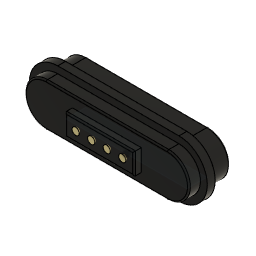
4pin_magnetic_connector_male v5 (Autodesk Fusion 360 design; units mm, degrees)
Autodesk Fusion 360 part; units mm, degrees
note: some values were not read from the file. Chosen so that the rebuilt part matches the saved one: which bodies a step acts on.
sketch "Skizze1" plane through (0, 0, 0) normal (0, 1, 0) x (1, 0, 0)
  line L0 (8.45, 3.95) -> (-8.45, 3.95)
  line L1 (-8.45, 3.95) -> (-8.45, -3.95)
  line L2 (-8.45, -3.95) -> (8.45, -3.95)
  line L3 (8.45, -3.95) -> (8.45, 3.95)
  line L4 (8.45, 3.95) -> (-8.45, -3.95) construction
  line L5 (-8.45, 3.95) -> (8.45, -3.95) construction
  arc A0 (8.45, -3.95) -> (8.45, 3.95) centre (8.45, 0) ccw
  arc A1 (-8.45, 3.95) -> (-8.45, -3.95) centre (-8.45, 0) ccw
  dimension "d1" = 16.9
  dimension "d2" = 7.9
  constraint horizontal L0
  constraint perpendicular L0 L1
  constraint parallel L0 L2
  constraint parallel L1 L3
  constraint coincident L4 origin
  constraint coincident L5 origin
  constraint midpoint L3 A0.centre
  constraint midpoint L1 A1.centre
  measures "d1" distance of L1.end L2.end
  measures "d2" distance of L0.end L1.end
extrude "Extrusion1" add sketch "Skizze1" along normal blind 1.1 makes body 1
sketch "Skizze2" plane through (0, 0, 0) normal (0, -1, 0) x (1, 0, 0)
  arc A0 (-8.45, 3.95) -> (-8.45, -3.95) centre (-8.45, 0) ccw
  line L0 (-8.45, -3.95) -> (8.45, -3.95)
  arc A1 (8.45, -3.95) -> (8.45, 3.95) centre (8.45, 0) ccw
  line L1 (8.45, 3.95) -> (-8.45, 3.95)
  arc A2 (-8.45, 3) -> (-8.45, -3) centre (-8.45, 0) ccw
  line L2 (-8.45, -3) -> (8.45, -3)
  arc A3 (8.45, -3) -> (8.45, 3) centre (8.45, 0) ccw
  line L3 (8.45, 3) -> (-8.45, 3)
  dimension "d5" = -0.95
extrude "Extrusion2" add sketch "Skizze2" along normal blind 1.6 contours A2 L2 A3 L3 bodies 1
sketch "Skizze3" plane through (0, 1.1, 0) normal (0, 1, 0) x (-1, 0, 0)
  arc A0 (8.45, -3.95) -> (8.45, 3.95) centre (8.45, 0) ccw
  line L0 (8.45, 3.95) -> (-8.45, 3.95)
  arc A1 (-8.45, 3.95) -> (-8.45, -3.95) centre (-8.45, 0) ccw
  line L1 (-8.45, -3.95) -> (8.45, -3.95)
  line L2 (-8.45, 3) -> (8.45, 3)
  arc A2 (8.45, -3) -> (8.45, 3) centre (8.45, 0) ccw
  line L3 (8.45, -3) -> (-8.45, -3)
  arc A3 (-8.45, 3) -> (-8.45, -3) centre (-8.45, 0) ccw
extrude "Extrusion3" add sketch "Skizze3" along normal blind 3 contours L2 A2 L3 A3 bodies 1
sketch "Skizze4" plane through (0, -1.6, 0) normal (0, -1, 0) x (1, 0, 0)
  line L0 (8.45, 3) -> (-8.45, 3)
  arc A0 (-8.45, 3) -> (-8.45, -3) centre (-8.45, 0) ccw
  line L1 (-8.45, -3) -> (8.45, -3)
  arc A1 (8.45, -3) -> (8.45, 3) centre (8.45, 0) ccw
  line L2 (4.8, -1.5) -> (-4.8, -1.5)
  line L3 (-4.8, -1.5) -> (-4.8, 1.5)
  line L4 (-4.8, 1.5) -> (4.8, 1.5)
  line L5 (4.8, 1.5) -> (4.8, -1.5)
  line L6 (4.8, -1.5) -> (-4.8, 1.5) construction
  line L7 (-4.8, -1.5) -> (4.8, 1.5) construction
  dimension "d10" = 9.6
  dimension "d11" = 3
  constraint horizontal L2
  constraint perpendicular L2 L3
  constraint parallel L2 L4
  constraint parallel L3 L5
  constraint coincident L6 origin
  constraint coincident L7 origin
  measures "d10" distance of L3.end L4.end
  measures "d11" distance of L2.end L3.end
extrude "Extrusion4" add sketch "Skizze4" along normal blind 1 contours L2 L3 L4 L5 bodies 1
sketch "Skizze5" plane through (0, -2.6, 0) normal (0, -1, 0) x (1, 0, 0)
  line L0 (4.8, 1.5) -> (-4.8, 1.5)
  line L1 (-4.8, 1.5) -> (-4.8, -1.5)
  line L2 (-4.8, -1.5) -> (4.8, -1.5)
  line L3 (4.8, -1.5) -> (4.8, 1.5)
  line L4 (-4.8, 0) -> (4.8, 0) construction
  circle A0 centre (-3.25, 0) radius 0.5
  circle A1 centre (-1.0833, 0) radius 0.5
  circle A2 centre (1.0833, 0) radius 0.5
  circle A3 centre (3.25, 0) radius 0.5
  line L5 (-3.25, 0) -> (-4.8, 0)
  line L6 (3.25, 0) -> (4.8, 0)
  dimension "d14" = 1
  dimension "d17" = 6.5
  dimension "d18" = 0
  constraint midpoint L1 L4.start
  constraint midpoint L3 L4.end
  constraint coincident L4 A0.centre
  constraint coincident A0.centre L5.start
  constraint perpendicular L1 L5
  constraint coincident A3.centre L6.start
  constraint perpendicular L3 L6
  constraint equal L5 L6
  measures "d14" diameter of A0
extrude "Extrusion5" add sketch "Skizze5" along normal blind 0.5 and the other way blind 8 separate body contours A0 | A1 | A2 | A3 makes body 2 at (-0.584, 2.7333, -0.0249) makes body 3 at (1.5827, 2.7333, -0.0249) makes body 4 at (-3.7494, 0.0667, -0.0249) makes body 5 at (3.7494, 2.7333, -0.0249)
fillet "Abrundung1" radius 0.2 12 edges at (0, -2.6, 1.5) (4.8, -2.6, 0) (0, -2.6, -1.5) (-4.8, -2.6, 0) (0, -1.6, -3) (11.45, -1.6, 0) (0, -1.6, 3) (-11.45, -1.6, 0) (0, 4.1, -3) (-11.45, 4.1, 0) (0, 4.1, 3) (11.45, 4.1, 0) on bodies 1
extrude "Extrusion6" cut 4 faces at (-3.1123, -3.1, 0.0939) (-1.1598, -3.1, 0.3624) (1.3465, -3.1, -0.1794) (3.3722, -3.1, 0.163) along direction (0, 1, 0) blind 0.4 on bodies 2 3 4 5 bodies 2 3 4 5
sketch "Skizze6" plane through (0, 0, -3) normal (0, 0, -1) x (1, 0, 0)
  line L0 (-8.45, -3.9) -> (8.45, -3.9)
  line L1 (8.45, -3.9) -> (8.45, -1.1)
  line L2 (8.45, -1.1) -> (-8.45, -1.1)
  line L3 (-8.45, -1.1) -> (-8.45, -3.9)
  point P0 (0, -1.1)
  constraint midpoint L2 P0
equation "d1 = 24.9 mm - 8 mm"
equation "d5 = -( 8 mm - 6.1 mm ) / 2"
